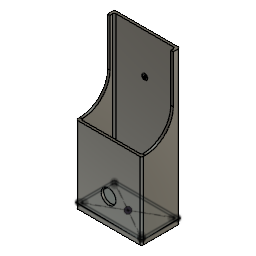
remote-holder v5 (Autodesk Fusion 360 design; units mm, degrees)
Autodesk Fusion 360 part; units mm, degrees
sketch "Sketch1" plane through (0, 0, 0) normal (0, 1, 0) x (1, 0, 0)
  line L0 (17.4, 44.65) -> (-17.4, 44.65)
  line L1 (-17.4, 44.65) -> (-17.4, -44.65)
  line L2 (-17.4, -44.65) -> (17.4, -44.65)
  line L3 (17.4, -44.65) -> (17.4, 44.65)
  line L4 (17.4, 44.65) -> (-17.4, -44.65) construction
  line L5 (-17.4, 44.65) -> (17.4, -44.65) construction
  dimension "d1" = 34.8
  dimension "d2" = 89.3
  constraint horizontal L0
  constraint perpendicular L0 L1
  constraint parallel L0 L2
  constraint parallel L1 L3
  constraint coincident L4 origin
  constraint coincident L5 origin
  measures "d1" distance of L1.end L2.end
  measures "d2" distance of L0.end L1.end
sketch "Sketch2" plane through (0, 0, 0) normal (0, 0, 1) x (1, 0, 0)
  line L0 (17.4, -10.15) -> (-17.4, -10.15)
  line L1 (-18.4, -9.15) -> (-18.4, 9.15)
  line L2 (-17.4, 10.15) -> (17.4, 10.15)
  line L3 (18.4, 9.15) -> (18.4, -9.15)
  line L4 (18.4, -10.15) -> (-18.4, 10.15) construction
  line L5 (-18.4, -10.15) -> (18.4, 10.15) construction
  line L6 (18.9, -11.65) -> (-18.9, -11.65)
  line L7 (-19.9, -10.65) -> (-19.9, 10.65)
  line L8 (-18.9, 11.65) -> (18.9, 11.65)
  line L9 (19.9, 10.65) -> (19.9, -10.65)
  line L10 (19.9, -11.65) -> (-19.9, 11.65) construction
  line L11 (-19.9, -11.65) -> (19.9, 11.65) construction
  arc A0 (-17.4, 10.15) -> (-18.4, 9.15) centre (-17.4, 9.15) ccw
  arc A1 (18.4, 9.15) -> (17.4, 10.15) centre (17.4, 9.15) ccw
  arc A2 (17.4, -10.15) -> (18.4, -9.15) centre (17.4, -9.15) ccw
  arc A3 (-18.4, -9.15) -> (-17.4, -10.15) centre (-17.4, -9.15) ccw
  arc A4 (-18.9, 11.65) -> (-19.9, 10.65) centre (-18.9, 10.65) ccw
  arc A5 (19.9, 10.65) -> (18.9, 11.65) centre (18.9, 10.65) ccw
  arc A6 (18.9, -11.65) -> (19.9, -10.65) centre (18.9, -10.65) ccw
  arc A7 (-19.9, -10.65) -> (-18.9, -11.65) centre (-18.9, -10.65) ccw
  dimension "d3" = 36.8
  dimension "d4" = 20.3
  dimension "d5" = 39.8
  dimension "d6" = 23.3
  dimension "d7" = 1
  dimension "d8" = 1
  constraint horizontal L0
  constraint perpendicular L0 L1
  constraint parallel L0 L2
  constraint parallel L1 L3
  constraint coincident L4 origin
  constraint coincident L5 origin
  constraint horizontal L6
  constraint perpendicular L6 L7
  constraint parallel L6 L8
  constraint parallel L7 L9
  constraint coincident L10 origin
  constraint coincident L11 origin
  constraint coincident L4.end L1
  constraint coincident L4.end L2
  constraint tangent L1 A0
  constraint tangent L2 A0
  constraint coincident L5.end L2
  constraint coincident L5.end L3
  constraint tangent L2 A1
  constraint tangent L3 A1
  constraint equal A0 A1
  constraint coincident L4.start L3
  constraint coincident L4.start L0
  constraint tangent L3 A2
  constraint tangent L0 A2
  constraint equal A0 A2
  constraint coincident L5.start L0
  constraint coincident L5.start L1
  constraint tangent L0 A3
  constraint tangent L1 A3
  constraint equal A0 A3
  constraint coincident L10.end L7
  constraint coincident L10.end L8
  constraint tangent L7 A4
  constraint tangent L8 A4
  constraint coincident L11.end L8
  constraint coincident L11.end L9
  constraint tangent L8 A5
  constraint tangent L9 A5
  constraint equal A4 A5
  constraint coincident L10.start L9
  constraint coincident L10.start L6
  constraint tangent L9 A6
  constraint tangent L6 A6
  constraint equal A4 A6
  constraint coincident L11.start L6
  constraint coincident L11.start L7
  constraint tangent L6 A7
  constraint tangent L7 A7
  constraint equal A4 A7
  measures "d3" distance of L4.end L5.end
  measures "d4" distance of L5.start L4.end
  measures "d5" distance of L10.end L11.end
  measures "d6" distance of L11.start L10.end
  measures "d7" radius of A0
  measures "d8" radius of A4
extrude "Extrude1" add sketch "Sketch2" along normal blind 89.3 makes body 1
extrude "Extrude2" add sketch "Sketch2" against normal blind 3 separate body contours L0 L1 L2 L3 A0 A1 A2 A3 | L6 L7 L8 L9 A4 A5 A6 A7 makes body 2
sketch "Sketch3" plane through (0, 0, 0) normal (1, 0, 0) x (0, 1, 0)
  line L0 (7.5, 94.5) -> (-22, 94.5)
  line L1 (-22, 94.5) -> (-22, 43.5)
  line L2 (-22, 43.5) -> (-9.5, 43.5)
  line L3 (7.5, 60.5) -> (7.5, 94.5)
  line L4 (-10.65, 0) -> (10.65, 0)
  arc A0 (-9.5, 43.5) -> (7.5, 60.5) centre (-9.5, 60.5) ccw
  dimension "d13" = 43.5
  dimension "d14" = 17
  constraint horizontal L0
  constraint vertical L1
  constraint horizontal L2
  constraint vertical L3
  constraint tangent L3 A0
  constraint tangent L2 A0
  measures "d13" distance of L2 L4
  measures "d14" radius of A0
extrude "Extrude3" cut sketch "Sketch3" along normal mid plane 200 bodies 1
hole "Hole1" at (-0.0142, 10.15, 64.9207) direction (0, 1, 0) diameter 1.8 depth 1 tip angle 118 counterbore diameter 3.5 counterbore depth 0.45 bodies 1
hole "Hole2" at (-0.0612, 10.15, 12.7709) direction (0, 1, 0) diameter 1.8 depth 1 tip angle 118 counterbore diameter 3.5 counterbore depth 0.45 bodies 1
hole "Hole3" at (-0.1501, -11.65, 12.9707) direction (0, 1, 0) diameter 9 depth 3 tip angle 180 bodies 1
combine "Combine1" operation add target body 1 tool bodies 2
equation "d5 = 36.8 mm + 3 mm"
equation "d6 = 20.3 mm + 3 mm"
